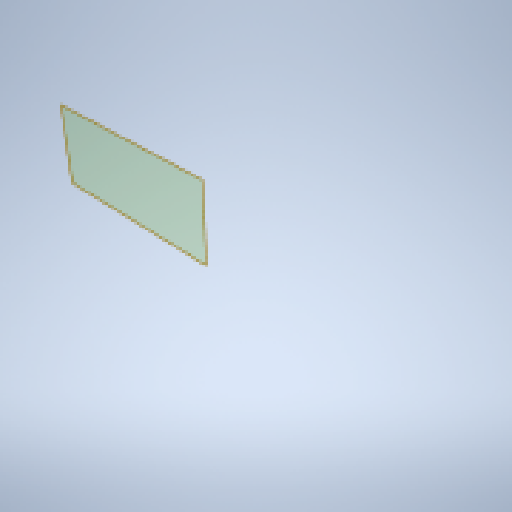
# Autodesk Inventor part: Part26
Saved by Autodesk Inventor 2023 (Build 270158000, 158)
## iProperties
Created: 2023-02-13
Part Number: Part26
Material: Generic
Document SubType Name: Modeling
Designer: klebe
Density: 1 g/cm^3
Appearance: Default
Author: klebe
Autodesk Inventor part; units mm, degrees
ref_plane "YZ Plane" through (0, 0, 0) normal (1, 0, 0) x (0, 1, 0)
ref_plane "XZ Plane" through (0, 0, 0) normal (0, 1, 0) x (-1, 0, 0)
ref_plane "XY Plane" through (0, 0, 0) normal (0, 0, 1) x (1, 0, 0)
ref_plane "Work Plane1" through (0, 0, -806) normal (0, 0, -1) x (-1, 0, 0)
sketch "Sketch1" plane through (0, 0, -806) normal (0, 0, -1) x (-1, 0, 0)
  line L0 (428.0132, 10) -> (663.0132, 10) projected
  line L1 (663.0132, 10) -> (663.0132, 110) projected
  line L2 (663.0132, 110) -> (428.0132, 110) projected
  line L3 (428.0132, 110) -> (428.0132, 10) projected
  point P0 (0, 0)
extrude "Extrusion1" add sketch "Sketch1" along normal blind 50
sketch "Sketch2" plane through (-663.0132, 110, -806) normal (0, 1, 0) x (1, 0, 0)
  line L0 (117.5, 50) -> (147.5, 50)
  line L1 (0, 0) -> (235, 0) projected
  line L2 (147.5, 50) -> (87.5, 50)
  line L3 (87.5, 50) -> (87.5, 0)
  line L4 (87.5, 0) -> (147.5, 0)
  line L5 (147.5, 0) -> (147.5, 50)
  point P0 (663.0132, -806)
  dimension "d4" = 60
  constraints: 10 end point, 2 parallel, 1 horizontal, 1 perpendicular, 1 point on line
  measures "d4" distance of L4.end L3.end
extrude "Extrusion2" add sketch "Sketch2" along normal blind 500
sketch "Sketch3" plane through (0, 0, -806) normal (0, 0, 1) x (1, 0, 0)
  line L0 (-663.0132, 10) -> (-663.0132, 110) projected
  line L1 (-428.0132, 10) -> (-663.0132, 10) projected
  line L2 (-428.0132, 110) -> (-428.0132, 10) projected
  line L3 (-515.5132, 110) -> (-428.0132, 110) projected
  line L4 (-515.5132, 110) -> (-515.5132, 610) projected
  line L5 (-575.5132, 610) -> (-515.5132, 610) projected
  line L6 (-575.5132, 110) -> (-575.5132, 610) projected
  line L7 (-663.0132, 110) -> (-575.5132, 110) projected
  line L8 (-575.5132, 110) -> (-575.5132, 610) projected
  line L9 (-515.5132, 110) -> (-515.5132, 610) projected
  line L10 (-575.5132, 610) -> (-515.5132, 610)
  line L11 (-515.5132, 610) -> (-515.5132, 550)
  line L12 (-515.5132, 550) -> (-575.5132, 550)
  line L13 (-575.5132, 550) -> (-575.5132, 610)
  point P0 (0, 0)
  dimension "d7" = 60
  constraints: 8 end point, 2 parallel, 1 horizontal, 1 perpendicular, 1 point on line
  measures "d7" distance of L10.end L11.end
extrude "Extrusion3" add sketch "Sketch3" along normal blind 300 contours L6 L5 L4 L12
sketch "Sketch4" plane through (-663.0132, 610, -806) normal (0, 1, 0) x (1, 0, 0)
  point P0 (663.0132, -806)
body "Solid1"
